Autodesk Fusion 360 part; units mm, degrees
(part 3 of 4)
  spline S28 degree 5 poles (-18.740221, -2.12836) (-18.744262, -2.124344) (-18.752452, -2.116435) (-18.765064, -2.104938) (-18.7825, -2.090307) (-18.805153, -2.072976) (-18.828436, -2.056341) (-18.852124, -2.040142) (-18.876048, -2.024187) (-18.90014, -2.008402) (-18.924398, -1.992794) (-18.948863, -1.977417) (-18.97359, -1.962339) (-18.998615, -1.947611) (-19.023939, -1.933234) (-19.049539, -1.919186) (-19.07538, -1.905425) (-19.101424, -1.891908) (-19.127643, -1.878606) (-19.154027, -1.865507) (-19.180576, -1.852613) (-19.207297, -1.839936) (-19.234197, -1.827485) (-19.261279, -1.815266) (-19.288542, -1.803279) (-19.315977, -1.791517) (-19.343576, -1.77997) (-19.37133, -1.768629) (-19.399233, -1.757488) (-19.427279, -1.746544) (-19.455469, -1.735796) (-19.4838, -1.725244) (-19.512273, -1.71489) (-19.540886, -1.704733) (-19.569636, -1.694772) (-19.598522, -1.685005) (-19.627539, -1.675429) (-19.656685, -1.666042) (-19.685956, -1.656842) (-19.71535, -1.647826) (-19.744866, -1.638995) (-19.774502, -1.630347) (-19.804256, -1.621883) (-19.834128, -1.613601) (-19.864114, -1.605501) (-19.894214, -1.597581) (-19.924425, -1.589841) (-19.954746, -1.582279) (-19.985174, -1.574894) (-20.015709, -1.567686) (-20.046348, -1.560654) (-20.077091, -1.553798) (-20.107936, -1.547117) (-20.138882, -1.540609) (-20.169926, -1.534276) (-20.201068, -1.528116) (-20.232307, -1.522128) (-20.26364, -1.516313) (-20.295067, -1.510669) (-20.326587, -1.505196) (-20.358197, -1.499894) (-20.389898, -1.494761) (-20.421688, -1.489799) (-20.453565, -1.485006) (-20.485528, -1.480381) (-20.517577, -1.475926) (-20.549708, -1.471638) (-20.581922, -1.467519) (-20.614218, -1.463567) (-20.646594, -1.459782) (-20.67905, -1.456164) (-20.705078, -1.453402) (-20.724635, -1.451406) (-20.737689, -1.450109) (-20.74422, -1.449468) knots 0 0 0 0 0 0 0.01428571 0.02857143 0.04285714 0.05714286 0.07142857 0.08571429 0.1 0.11428571 0.12857143 0.14285714 0.15714286 0.17142857 0.18571429 0.2 0.21428571 0.22857143 0.24285714 0.25714286 0.27142857 0.28571429 0.3 0.31428571 0.32857143 0.34285714 0.35714286 0.37142857 0.38571429 0.4 0.41428571 0.42857143 0.44285714 0.45714286 0.47142857 0.48571429 0.5 0.51428571 0.52857143 0.54285714 0.55714286 0.57142857 0.58571429 0.6 0.61428571 0.62857143 0.64285714 0.65714286 0.67142857 0.68571429 0.7 0.71428571 0.72857143 0.74285714 0.75714286 0.77142857 0.78571429 0.8 0.81428571 0.82857143 0.84285714 0.85714286 0.87142857 0.88571429 0.9 0.91428571 0.92857143 0.94285714 0.95714286 0.97142857 0.98571429 1 1 1 1 1 1
  arc A14 (-20.74422, -1.449468) -> (-21.063932, -1.847201) centre (-12.332883, -8.53815) ccw
  spline S29 degree 5 poles (-19.970136, -3.658422) (-19.974927, -3.655338) (-19.984412, -3.649039) (-19.998351, -3.639194) (-20.016388, -3.62531) (-20.038183, -3.606913) (-20.059434, -3.58775) (-20.080347, -3.568098) (-20.101071, -3.548162) (-20.121666, -3.528027) (-20.142123, -3.507691) (-20.1624, -3.487103) (-20.18244, -3.466195) (-20.202204, -3.444921) (-20.221688, -3.42328) (-20.240911, -3.401298) (-20.259905, -3.379019) (-20.278704, -3.35649) (-20.297331, -3.333743) (-20.315796, -3.310791) (-20.334094, -3.287634) (-20.352219, -3.264263) (-20.370162, -3.240669) (-20.387916, -3.216846) (-20.405483, -3.192797) (-20.422868, -3.168532) (-20.440078, -3.14406) (-20.457119, -3.119392) (-20.473997, -3.094537) (-20.490715, -3.069498) (-20.507271, -3.044278) (-20.523667, -3.018877) (-20.539899, -2.993296) (-20.555969, -2.967535) (-20.571877, -2.941598) (-20.587625, -2.915487) (-20.603214, -2.889206) (-20.618647, -2.86276) (-20.633925, -2.836151) (-20.649048, -2.809382) (-20.664017, -2.782454) (-20.678833, -2.75537) (-20.693495, -2.72813) (-20.708005, -2.700738) (-20.722361, -2.673193) (-20.736566, -2.6455) (-20.75062, -2.617659) (-20.764523, -2.589672) (-20.778276, -2.561543) (-20.791879, -2.533271) (-20.805332, -2.504859) (-20.818637, -2.476309) (-20.831792, -2.447621) (-20.844799, -2.418798) (-20.857658, -2.38984) (-20.870368, -2.36075) (-20.882931, -2.331529) (-20.895345, -2.302178) (-20.907613, -2.272699) (-20.919733, -2.243093) (-20.931707, -2.213361) (-20.943533, -2.183505) (-20.955213, -2.153525) (-20.966747, -2.123423) (-20.978134, -2.093201) (-20.989374, -2.06286) (-21.000468, -2.032401) (-21.011416, -2.001825) (-21.022218, -1.971134) (-21.032874, -1.940329) (-21.043384, -1.909409) (-21.051675, -1.884583) (-21.057829, -1.865912) (-21.061902, -1.853442) (-21.063932, -1.847201) knots 0 0 0 0 0 0 0.01428571 0.02857143 0.04285714 0.05714286 0.07142857 0.08571429 0.1 0.11428571 0.12857143 0.14285714 0.15714286 0.17142857 0.18571429 0.2 0.21428571 0.22857143 0.24285714 0.25714286 0.27142857 0.28571429 0.3 0.31428571 0.32857143 0.34285714 0.35714286 0.37142857 0.38571429 0.4 0.41428571 0.42857143 0.44285714 0.45714286 0.47142857 0.48571429 0.5 0.51428571 0.52857143 0.54285714 0.55714286 0.57142857 0.58571429 0.6 0.61428571 0.62857143 0.64285714 0.65714286 0.67142857 0.68571429 0.7 0.71428571 0.72857143 0.74285714 0.75714286 0.77142857 0.78571429 0.8 0.81428571 0.82857143 0.84285714 0.85714286 0.87142857 0.88571429 0.9 0.91428571 0.92857143 0.94285714 0.95714286 0.97142857 0.98571429 1 1 1 1 1 1
  line L29 (-19.970136, -3.658422) -> (-19.69789, -3.833648)
  line L30 (-20.118424, -4.568134) -> (-20.407357, -4.422054)
  spline S30 degree 5 poles (-20.407357, -4.422054) (-20.412442, -4.419483) (-20.422675, -4.414492) (-20.438222, -4.407455) (-20.459326, -4.398929) (-20.486226, -4.389446) (-20.51351, -4.380819) (-20.541045, -4.372733) (-20.568728, -4.364952) (-20.596518, -4.357385) (-20.624412, -4.350037) (-20.652432, -4.342972) (-20.680608, -4.336273) (-20.708959, -4.329999) (-20.737487, -4.324152) (-20.766175, -4.318702) (-20.795003, -4.313599) (-20.823949, -4.308793) (-20.852996, -4.304243) (-20.882136, -4.299938) (-20.91137, -4.29588) (-20.940701, -4.29208) (-20.970132, -4.288551) (-20.999665, -4.2853) (-21.029297, -4.282324) (-21.059024, -4.279615) (-21.088841, -4.277162) (-21.118741, -4.274953) (-21.14872, -4.27298) (-21.178777, -4.271238) (-21.208908, -4.269726) (-21.239113, -4.268446) (-21.269392, -4.267397) (-21.299743, -4.266579) (-21.330164, -4.265991) (-21.360655, -4.265628) (-21.391211, -4.265487) (-21.42183, -4.265566) (-21.452512, -4.265861) (-21.483254, -4.26637) (-21.514054, -4.267092) (-21.544911, -4.268026) (-21.575825, -4.269171) (-21.606794, -4.270525) (-21.637816, -4.272087) (-21.66889, -4.273856) (-21.700014, -4.27583) (-21.731187, -4.278008) (-21.762409, -4.280388) (-21.793676, -4.282969) (-21.824989, -4.285749) (-21.856346, -4.288728) (-21.887746, -4.291906) (-21.919188, -4.29528) (-21.95067, -4.29885) (-21.982192, -4.302614) (-22.013751, -4.306573) (-22.045348, -4.310725) (-22.076981, -4.315069) (-22.108649, -4.319604) (-22.140351, -4.324329) (-22.172086, -4.329244) (-22.203854, -4.334348) (-22.235652, -4.33964) (-22.26748, -4.345119) (-22.299336, -4.350785) (-22.33122, -4.356636) (-22.363131, -4.362673) (-22.395067, -4.368895) (-22.427028, -4.3753) (-22.459013, -4.381888) (-22.484621, -4.387305) (-22.503838, -4.39145) (-22.516654, -4.39425) (-22.523063, -4.395659) knots 0 0 0 0 0 0 0.01428571 0.02857143 0.04285714 0.05714286 0.07142857 0.08571429 0.1 0.11428571 0.12857143 0.14285714 0.15714286 0.17142857 0.18571429 0.2 0.21428571 0.22857143 0.24285714 0.25714286 0.27142857 0.28571429 0.3 0.31428571 0.32857143 0.34285714 0.35714286 0.37142857 0.38571429 0.4 0.41428571 0.42857143 0.44285714 0.45714286 0.47142857 0.48571429 0.5 0.51428571 0.52857143 0.54285714 0.55714286 0.57142857 0.58571429 0.6 0.61428571 0.62857143 0.64285714 0.65714286 0.67142857 0.68571429 0.7 0.71428571 0.72857143 0.74285714 0.75714286 0.77142857 0.78571429 0.8 0.81428571 0.82857143 0.84285714 0.85714286 0.87142857 0.88571429 0.9 0.91428571 0.92857143 0.94285714 0.95714286 0.97142857 0.98571429 1 1 1 1 1 1
  arc A15 (-22.523063, -4.395659) -> (-22.70422, -4.872722) centre (-12.332883, -8.53815) ccw
  spline S31 degree 5 poles (-21.104261, -6.257294) (-21.10977, -6.255842) (-21.120737, -6.252782) (-21.137036, -6.247726) (-21.158481, -6.240095) (-21.184895, -6.229333) (-21.211028, -6.217675) (-21.236989, -6.205447) (-21.26286, -6.192892) (-21.288668, -6.180106) (-21.314409, -6.167087) (-21.340056, -6.153773) (-21.365576, -6.140081) (-21.390946, -6.125956) (-21.416164, -6.111394) (-21.441239, -6.096428) (-21.466188, -6.081109) (-21.491029, -6.065492) (-21.515774, -6.049615) (-21.540427, -6.033492) (-21.564986, -6.017123) (-21.589446, -6.000497) (-21.613801, -5.983602) (-21.638048, -5.966431) (-21.662187, -5.948988) (-21.686219, -5.931282) (-21.710149, -5.913326) (-21.733979, -5.895132) (-21.757712, -5.876709) (-21.781348, -5.858062) (-21.804888, -5.839192) (-21.82833, -5.820101) (-21.851673, -5.800788) (-21.874917, -5.781254) (-21.898062, -5.761502) (-21.921108, -5.741535) (-21.944055, -5.721358) (-21.966905, -5.700975) (-21.989657, -5.68039) (-22.012312, -5.659604) (-22.03487, -5.63862) (-22.05733, -5.61744) (-22.079693, -5.596064) (-22.101957, -5.574496) (-22.124122, -5.552736) (-22.14619, -5.530788) (-22.168159, -5.508652) (-22.19003, -5.486332) (-22.211802, -5.463828) (-22.233475, -5.441144) (-22.25505, -5.41828) (-22.276526, -5.395238) (-22.297903, -5.37202) (-22.31918, -5.348627) (-22.340358, -5.32506) (-22.361435, -5.301322) (-22.382413, -5.277413) (-22.40329, -5.253335) (-22.424066, -5.229089) (-22.444742, -5.204678) (-22.465317, -5.180101) (-22.485791, -5.15536) (-22.506164, -5.130457) (-22.526435, -5.105393) (-22.546604, -5.080169) (-22.56667, -5.054786) (-22.586633, -5.029246) (-22.606494, -5.00355) (-22.626251, -4.977699) (-22.645905, -4.951694) (-22.665455, -4.925536) (-22.681013, -4.904486) (-22.692635, -4.888631) (-22.700362, -4.87803) (-22.70422, -4.872722) knots 0 0 0 0 0 0 0.01428571 0.02857143 0.04285714 0.05714286 0.07142857 0.08571429 0.1 0.11428571 0.12857143 0.14285714 0.15714286 0.17142857 0.18571429 0.2 0.21428571 0.22857143 0.24285714 0.25714286 0.27142857 0.28571429 0.3 0.31428571 0.32857143 0.34285714 0.35714286 0.37142857 0.38571429 0.4 0.41428571 0.42857143 0.44285714 0.45714286 0.47142857 0.48571429 0.5 0.51428571 0.52857143 0.54285714 0.55714286 0.57142857 0.58571429 0.6 0.61428571 0.62857143 0.64285714 0.65714286 0.67142857 0.68571429 0.7 0.71428571 0.72857143 0.74285714 0.75714286 0.77142857 0.78571429 0.8 0.81428571 0.82857143 0.84285714 0.85714286 0.87142857 0.88571429 0.9 0.91428571 0.92857143 0.94285714 0.95714286 0.97142857 0.98571429 1 1 1 1 1 1
  line L31 (-21.104261, -6.257294) -> (-20.791192, -6.339815)
  line L32 (-20.964175, -7.168305) -> (-21.284108, -7.11866)
  spline S32 degree 5 poles (-21.284108, -7.11866) (-21.289738, -7.117786) (-21.301013, -7.116202) (-21.317973, -7.114314) (-21.34068, -7.112726) (-21.369193, -7.112019) (-21.397807, -7.112246) (-21.426493, -7.113065) (-21.455226, -7.114219) (-21.483995, -7.11561) (-21.512794, -7.117241) (-21.541626, -7.119181) (-21.570492, -7.121517) (-21.599395, -7.12431) (-21.628333, -7.127565) (-21.657302, -7.131247) (-21.686296, -7.135303) (-21.71531, -7.139676) (-21.744341, -7.144325) (-21.773385, -7.149236) (-21.802443, -7.15441) (-21.831512, -7.15986) (-21.860593, -7.165598) (-21.889685, -7.171632) (-21.918786, -7.177959) (-21.947896, -7.184569) (-21.977011, -7.191449) (-22.006131, -7.198588) (-22.035253, -7.205975) (-22.064376, -7.213607) (-22.093499, -7.22148) (-22.122622, -7.229597) (-22.151743, -7.237956) (-22.180861, -7.246557) (-22.209976, -7.255398) (-22.239086, -7.264475) (-22.26819, -7.273784) (-22.297287, -7.283321) (-22.326375, -7.293082) (-22.355455, -7.303066) (-22.384525, -7.313271) (-22.413583, -7.323694) (-22.442631, -7.334335) (-22.471665, -7.345193) (-22.500686, -7.356265) (-22.529692, -7.36755) (-22.558683, -7.379046) (-22.587658, -7.39075) (-22.616616, -7.402661) (-22.645555, -7.414778) (-22.674477, -7.427099) (-22.703378, -7.439622) (-22.732259, -7.452347) (-22.76112, -7.465272) (-22.789958, -7.478395) (-22.818773, -7.491717) (-22.847565, -7.505234) (-22.876333, -7.518947) (-22.905075, -7.532853) (-22.933792, -7.546952) (-22.962482, -7.561242) (-22.991145, -7.575723) (-23.01978, -7.590394) (-23.048387, -7.605253) (-23.076964, -7.6203) (-23.10551, -7.635532) (-23.134026, -7.65095) (-23.162509, -7.666553) (-23.190959, -7.682338) (-23.219377, -7.698306) (-23.247761, -7.714456) (-23.270441, -7.727522) (-23.287437, -7.737402) (-23.29876, -7.744025) (-23.30442, -7.747346) knots 0 0 0 0 0 0 0.01428571 0.02857143 0.04285714 0.05714286 0.07142857 0.08571429 0.1 0.11428571 0.12857143 0.14285714 0.15714286 0.17142857 0.18571429 0.2 0.21428571 0.22857143 0.24285714 0.25714286 0.27142857 0.28571429 0.3 0.31428571 0.32857143 0.34285714 0.35714286 0.37142857 0.38571429 0.4 0.41428571 0.42857143 0.44285714 0.45714286 0.47142857 0.48571429 0.5 0.51428571 0.52857143 0.54285714 0.55714286 0.57142857 0.58571429 0.6 0.61428571 0.62857143 0.64285714 0.65714286 0.67142857 0.68571429 0.7 0.71428571 0.72857143 0.74285714 0.75714286 0.77142857 0.78571429 0.8 0.81428571 0.82857143 0.84285714 0.85714286 0.87142857 0.88571429 0.9 0.91428571 0.92857143 0.94285714 0.95714286 0.97142857 0.98571429 1 1 1 1 1 1
  arc A16 (-23.30442, -7.747346) -> (-23.329291, -8.25704) centre (-12.332883, -8.53815) ccw
  spline S33 degree 5 poles (-21.379783, -9.079432) (-21.385471, -9.079753) (-21.396847, -9.080232) (-21.41391, -9.08046) (-21.436663, -9.07983) (-21.46511, -9.077757) (-21.493566, -9.074745) (-21.522036, -9.071138) (-21.55052, -9.067192) (-21.579017, -9.063007) (-21.607521, -9.058579) (-21.636026, -9.053842) (-21.664528, -9.048707) (-21.693022, -9.043112) (-21.721506, -9.037056) (-21.749978, -9.030571) (-21.778439, -9.023712) (-21.80689, -9.016535) (-21.835331, -9.009081) (-21.863759, -9.001366) (-21.892175, -8.993387) (-21.920575, -8.985134) (-21.948959, -8.976591) (-21.977326, -8.967754) (-22.005673, -8.958624) (-22.034001, -8.949211) (-22.062308, -8.939529) (-22.090594, -8.929589) (-22.118858, -8.919401) (-22.1471, -8.908971) (-22.175319, -8.898299) (-22.203513, -8.887386) (-22.231682, -8.876232) (-22.259824, -8.864837) (-22.28794, -8.853203) (-22.316028, -8.841335) (-22.344087, -8.829237) (-22.372117, -8.816913) (-22.400118, -8.804366) (-22.428087, -8.791598) (-22.456025, -8.778612) (-22.483931, -8.765409) (-22.511804, -8.75199) (-22.539644, -8.738357) (-22.567449, -8.724512) (-22.595218, -8.710457) (-22.622953, -8.696193) (-22.65065, -8.681724) (-22.678311, -8.66705) (-22.705933, -8.652173) (-22.733518, -8.637096) (-22.761063, -8.621818) (-22.788568, -8.606342) (-22.816033, -8.590669) (-22.843456, -8.5748) (-22.870838, -8.558736) (-22.898177, -8.54248) (-22.925473, -8.526032) (-22.952725, -8.509393) (-22.979932, -8.492566) (-23.007095, -8.47555) (-23.034212, -8.458347) (-23.061283, -8.440958) (-23.088307, -8.423385) (-23.115283, -8.405627) (-23.142211, -8.387688) (-23.16909, -8.369567) (-23.195919, -8.351266) (-23.222697, -8.332785) (-23.249425, -8.314127) (-23.276102, -8.29529) (-23.297403, -8.280078) (-23.313356, -8.26859) (-23.323981, -8.260896) (-23.329291, -8.25704) knots 0 0 0 0 0 0 0.01428571 0.02857143 0.04285714 0.05714286 0.07142857 0.08571429 0.1 0.11428571 0.12857143 0.14285714 0.15714286 0.17142857 0.18571429 0.2 0.21428571 0.22857143 0.24285714 0.25714286 0.27142857 0.28571429 0.3 0.31428571 0.32857143 0.34285714 0.35714286 0.37142857 0.38571429 0.4 0.41428571 0.42857143 0.44285714 0.45714286 0.47142857 0.48571429 0.5 0.51428571 0.52857143 0.54285714 0.55714286 0.57142857 0.58571429 0.6 0.61428571 0.62857143 0.64285714 0.65714286 0.67142857 0.68571429 0.7 0.71428571 0.72857143 0.74285714 0.75714286 0.77142857 0.78571429 0.8 0.81428571 0.82857143 0.84285714 0.85714286 0.87142857 0.88571429 0.9 0.91428571 0.92857143 0.94285714 0.95714286 0.97142857 0.98571429 1 1 1 1 1 1
  line L33 (-21.379783, -9.079432) -> (-21.056536, -9.06117)
  line L34 (-20.965034, -9.902566) -> (-21.284651, -9.954215)
  spline S34 degree 5 poles (-21.284651, -9.954215) (-21.290275, -9.955124) (-21.301487, -9.957101) (-21.318201, -9.960547) (-21.340287, -9.966053) (-21.367623, -9.974192) (-21.394767, -9.983251) (-21.421796, -9.992893) (-21.448766, -10.00287) (-21.475696, -10.013083) (-21.502582, -10.023534) (-21.529403, -10.034288) (-21.556135, -10.04543) (-21.58276, -10.057018) (-21.609276, -10.069056) (-21.635689, -10.081509) (-21.662011, -10.094326) (-21.688254, -10.107451) (-21.714427, -10.120844) (-21.740532, -10.13449) (-21.766569, -10.14839) (-21.792531, -10.162556) (-21.818416, -10.177) (-21.844219, -10.191728) (-21.869941, -10.206738) (-21.895583, -10.22202) (-21.921147, -10.237561) (-21.946636, -10.253349) (-21.972049, -10.269374) (-21.997389, -10.285631) (-22.022654, -10.302119) (-22.047843, -10.318837) (-22.072956, -10.335786) (-22.097991, -10.352965) (-22.122949, -10.37037) (-22.147829, -10.387998) (-22.172632, -10.405845) (-22.197357, -10.423906) (-22.222006, -10.442179) (-22.246577, -10.46066) (-22.271071, -10.479348) (-22.295486, -10.498242) (-22.319823, -10.517338) (-22.344081, -10.536637) (-22.36826, -10.556135) (-22.39236, -10.575831) (-22.41638, -10.595722) (-22.440319, -10.615807) (-22.464179, -10.636084) (-22.487958, -10.656551) (-22.511657, -10.677205) (-22.535274, -10.698047) (-22.558809, -10.719074) (-22.582263, -10.740284) (-22.605634, -10.761677) (-22.628923, -10.783251) (-22.652128, -10.805004) (-22.67525, -10.826935) (-22.698289, -10.849042) (-22.721243, -10.871325) (-22.744113, -10.893782) (-22.766899, -10.916412) (-22.789599, -10.939213) (-22.812214, -10.962185) (-22.834742, -10.985326) (-22.857185, -11.008635) (-22.87954, -11.03211) (-22.901808, -11.05575) (-22.923987, -11.079555) (-22.94608, -11.103523) (-22.968084, -11.127653) (-22.985617, -11.147088) (-22.998727, -11.161737) (-23.00745, -11.171535) (-23.011807, -11.176442) knots 0 0 0 0 0 0 0.01428571 0.02857143 0.04285714 0.05714286 0.07142857 0.08571429 0.1 0.11428571 0.12857143 0.14285714 0.15714286 0.17142857 0.18571429 0.2 0.21428571 0.22857143 0.24285714 0.25714286 0.27142857 0.28571429 0.3 0.31428571 0.32857143 0.34285714 0.35714286 0.37142857 0.38571429 0.4 0.41428571 0.42857143 0.44285714 0.45714286 0.47142857 0.48571429 0.5 0.51428571 0.52857143 0.54285714 0.55714286 0.57142857 0.58571429 0.6 0.61428571 0.62857143 0.64285714 0.65714286 0.67142857 0.68571429 0.7 0.71428571 0.72857143 0.74285714 0.75714286 0.77142857 0.78571429 0.8 0.81428571 0.82857143 0.84285714 0.85714286 0.87142857 0.88571429 0.9 0.91428571 0.92857143 0.94285714 0.95714286 0.97142857 0.98571429 1 1 1 1 1 1
  arc A17 (-23.011807, -11.176442) -> (-22.877956, -11.668875) centre (-12.332883, -8.53815) ccw
  spline S35 degree 5 poles (-20.769731, -11.848585) (-20.775041, -11.850648) (-20.785712, -11.854619) (-20.80187, -11.860109) (-20.823704, -11.866541) (-20.851399, -11.87336) (-20.879394, -11.879289) (-20.907585, -11.884656) (-20.935894, -11.889705) (-20.964289, -11.894531) (-20.992766, -11.899128) (-21.021341, -11.903431) (-21.050034, -11.907355) (-21.078862, -11.91084) (-21.107823, -11.913882) (-21.136906, -11.916513) (-21.166094, -11.918784) (-21.19537, -11.92075) (-21.224722, -11.92245) (-21.254143, -11.923897) (-21.283633, -11.92509) (-21.313195, -11.926016) (-21.342829, -11.926664) (-21.372538, -11.927024) (-21.402319, -11.927101) (-21.432169, -11.926903) (-21.462083, -11.926441) (-21.492056, -11.925729) (-21.522085, -11.924774) (-21.552168, -11.923582) (-21.582303, -11.922152) (-21.61249, -11.920486) (-21.642727, -11.918582) (-21.673014, -11.916441) (-21.703348, -11.914065) (-21.733728, -11.911458) (-21.764153, -11.908623) (-21.79462, -11.905563) (-21.825127, -11.902283) (-21.855673, -11.898783) (-21.886256, -11.895066) (-21.916877, -11.891132) (-21.947532, -11.886983) (-21.978222, -11.882621) (-22.008944, -11.878046) (-22.039698, -11.87326) (-22.070483, -11.868265) (-22.101296, -11.863062) (-22.132137, -11.857654) (-22.163005, -11.852042) (-22.193898, -11.846226) (-22.224816, -11.840208) (-22.255758, -11.833989) (-22.286722, -11.82757) (-22.317707, -11.820952) (-22.348712, -11.814136) (-22.379736, -11.807123) (-22.410779, -11.799915) (-22.441839, -11.792512) (-22.472915, -11.784916) (-22.504006, -11.777127) (-22.535112, -11.769145) (-22.566231, -11.760973) (-22.597363, -11.75261) (-22.628507, -11.744058) (-22.659661, -11.735318) (-22.690823, -11.72639) (-22.721995, -11.717275) (-22.753173, -11.707974) (-22.784359, -11.698488) (-22.815551, -11.688817) (-22.84051, -11.680932) (-22.859232, -11.674936) (-22.871714, -11.670902) (-22.877956, -11.668875) knots 0 0 0 0 0 0 0.01428571 0.02857143 0.04285714 0.05714286 0.07142857 0.08571429 0.1 0.11428571 0.12857143 0.14285714 0.15714286 0.17142857 0.18571429 0.2 0.21428571 0.22857143 0.24285714 0.25714286 0.27142857 0.28571429 0.3 0.31428571 0.32857143 0.34285714 0.35714286 0.37142857 0.38571429 0.4 0.41428571 0.42857143 0.44285714 0.45714286 0.47142857 0.48571429 0.5 0.51428571 0.52857143 0.54285714 0.55714286 0.57142857 0.58571429 0.6 0.61428571 0.62857143 0.64285714 0.65714286 0.67142857 0.68571429 0.7 0.71428571 0.72857143 0.74285714 0.75714286 0.77142857 0.78571429 0.8 0.81428571 0.82857143 0.84285714 0.85714286 0.87142857 0.88571429 0.9 0.91428571 0.92857143 0.94285714 0.95714286 0.97142857 0.98571429 1 1 1 1 1 1
  line L35 (-20.769731, -11.848585) -> (-20.467948, -11.731329)
  line L36 (-20.120919, -12.503268) -> (-20.408932, -12.651156)
  spline S36 degree 5 poles (-20.408932, -12.651156) (-20.413999, -12.653758) (-20.424053, -12.659104) (-20.438884, -12.667546) (-20.458187, -12.679607) (-20.48167, -12.695796) (-20.504686, -12.712798) (-20.527412, -12.730321) (-20.549979, -12.748144) (-20.572436, -12.766179) (-20.594776, -12.784427) (-20.616961, -12.802943) (-20.638942, -12.8218) (-20.660683, -12.841049) (-20.682181, -12.860691) (-20.703453, -12.880697) (-20.724526, -12.901021) (-20.745428, -12.921613) (-20.766182, -12.942438) (-20.786793, -12.963483) (-20.807259, -12.984748) (-20.827574, -13.006244) (-20.847728, -13.027979) (-20.867717, -13.049961) (-20.887542, -13.072185) (-20.907207, -13.094642) (-20.926717, -13.117323) (-20.946079, -13.140214) (-20.965297, -13.163308) (-20.984373, -13.1866) (-21.003306, -13.210088) (-21.022097, -13.233772) (-21.040743, -13.257652) (-21.059244, -13.281726) (-21.077602, -13.305991) (-21.095817, -13.330445) (-21.113891, -13.355083) (-21.131825, -13.379901) (-21.149621, -13.404896) (-21.167278, -13.430066) (-21.184798, -13.455408) (-21.20218, -13.480922) (-21.219425, -13.506604) (-21.236532, -13.532454) (-21.253502, -13.55847) (-21.270336, -13.584649) (-21.287033, -13.610989) (-21.303595, -13.637489) (-21.320021, -13.664147) (-21.336312, -13.69096) (-21.352467, -13.717927) (-21.368488, -13.745046) (-21.384374, -13.772317) (-21.400126, -13.799737) (-21.415742, -13.827305) (-21.431224, -13.855019) (-21.446572, -13.882878) (-21.461785, -13.910881) (-21.476865, -13.939026) (-21.49181, -13.967311) (-21.506621, -13.995736) (-21.521298, -14.024299) (-21.535841, -14.053) (-21.550251, -14.081836) (-21.564526, -14.110806) (-21.578667, -14.139908) (-21.592674, -14.169143) (-21.606546, -14.198507) (-21.620285, -14.228001) (-21.633889, -14.257622) (-21.647359, -14.287372) (-21.658029, -14.311273) (-21.665971, -14.329256) (-21.671239, -14.34127) (-21.673866, -14.347284) knots 0 0 0 0 0 0 0.01428571 0.02857143 0.04285714 0.05714286 0.07142857 0.08571429 0.1 0.11428571 0.12857143 0.14285714 0.15714286 0.17142857 0.18571429 0.2 0.21428571 0.22857143 0.24285714 0.25714286 0.27142857 0.28571429 0.3 0.31428571 0.32857143 0.34285714 0.35714286 0.37142857 0.38571429 0.4 0.41428571 0.42857143 0.44285714 0.45714286 0.47142857 0.48571429 0.5 0.51428571 0.52857143 0.54285714 0.55714286 0.57142857 0.58571429 0.6 0.61428571 0.62857143 0.64285714 0.65714286 0.67142857 0.68571429 0.7 0.71428571 0.72857143 0.74285714 0.75714286 0.77142857 0.78571429 0.8 0.81428571 0.82857143 0.84285714 0.85714286 0.87142857 0.88571429 0.9 0.91428571 0.92857143 0.94285714 0.95714286 0.97142857 0.98571429 1 1 1 1 1 1
  arc A18 (-21.673866, -14.347284) -> (-21.394396, -14.774253) centre (-12.332883, -8.53815) ccw
  spline S37 degree 5 poles (-19.333821, -14.29369) (-19.338234, -14.297293) (-19.347156, -14.304368) (-19.360827, -14.314582) (-19.379605, -14.327446) (-19.403837, -14.342489) (-19.428629, -14.356779) (-19.453782, -14.370595) (-19.479145, -14.384145) (-19.504659, -14.397509) (-19.530322, -14.410681) (-19.556168, -14.423604) (-19.582245, -14.436202) (-19.608585, -14.448425) (-19.635189, -14.460267) (-19.662035, -14.471757) (-19.689093, -14.482936) (-19.716328, -14.493853) (-19.743718, -14.50454) (-19.771252, -14.515008) (-19.79893, -14.525255) (-19.826759, -14.535271) (-19.854743, -14.545044) (-19.882886, -14.554568) (-19.911186, -14.563844) (-19.939636, -14.572879) (-19.968228, -14.581684) (-19.996955, -14.590269) (-20.025809, -14.598641) (-20.054788, -14.606803) (-20.08389, -14.614755) (-20.113114, -14.622499) (-20.14246, -14.630032) (-20.171926, -14.637355) (-20.20151, -14.644469) (-20.231209, -14.651377) (-20.26102, -14.658083) (-20.290941, -14.664588) (-20.320969, -14.670895) (-20.351102, -14.677006) (-20.381337, -14.682921) (-20.411674, -14.688642) (-20.442111, -14.69417) (-20.472647, -14.699504) (-20.503279, -14.704647) (-20.534007, -14.709598) (-20.564828, -14.714361) (-20.595741, -14.718935) (-20.626744, -14.723322) (-20.657836, -14.727523) (-20.689014, -14.731538) (-20.720279, -14.735369) (-20.751627, -14.739016) (-20.783059, -14.742479) (-20.814573, -14.74576) (-20.846167, -14.748859) (-20.87784, -14.751777) (-20.909591, -14.754514) (-20.941418, -14.757072) (-20.97332, -14.75945) (-21.005297, -14.76165) (-21.037347, -14.763671) (-21.069469, -14.765515) (-21.101661, -14.767182) (-21.133923, -14.768673) (-21.166253, -14.769987) (-21.198649, -14.771126) (-21.231111, -14.77209) (-21.263638, -14.772879) (-21.296229, -14.773494) (-21.328883, -14.773935) (-21.355056, -14.774149) (-21.374715, -14.774231) (-21.387833, -14.774252) (-21.394396, -14.774253) knots 0 0 0 0 0 0 0.01428571 0.02857143 0.04285714 0.05714286 0.07142857 0.08571429 0.1 0.11428571 0.12857143 0.14285714 0.15714286 0.17142857 0.18571429 0.2 0.21428571 0.22857143 0.24285714 0.25714286 0.27142857 0.28571429 0.3 0.31428571 0.32857143 0.34285714 0.35714286 0.37142857 0.38571429 0.4 0.41428571 0.42857143 0.44285714 0.45714286 0.47142857 0.48571429 0.5 0.51428571 0.52857143 0.54285714 0.55714286 0.57142857 0.58571429 0.6 0.61428571 0.62857143 0.64285714 0.65714286 0.67142857 0.68571429 0.7 0.71428571 0.72857143 0.74285714 0.75714286 0.77142857 0.78571429 0.8 0.81428571 0.82857143 0.84285714 0.85714286 0.87142857 0.88571429 0.9 0.91428571 0.92857143 0.94285714 0.95714286 0.97142857 0.98571429 1 1 1 1 1 1
  line L37 (-19.333821, -14.29369) -> (-19.083043, -14.088917)
  line L38 (-18.514457, -14.715837) -> (-18.742673, -14.945488)
  spline S38 degree 5 poles (-18.742673, -14.945488) (-18.746688, -14.949529) (-18.754598, -14.957719) (-18.766094, -14.970331) (-18.780725, -14.987767) (-18.798056, -15.01042) (-18.814692, -15.033703) (-18.830891, -15.057391) (-18.846846, -15.081315) (-18.862631, -15.105406) (-18.878239, -15.129665) (-18.893616, -15.15413) (-18.908694, -15.178856) (-18.923422, -15.203882) (-18.937799, -15.229206) (-18.951847, -15.254806) (-18.965608, -15.280647) (-18.979125, -15.30669) (-18.992427, -15.332909) (-19.005526, -15.359293) (-19.018419, -15.385843) (-19.031097, -15.412563) (-19.043548, -15.439463) (-19.055766, -15.466546) (-19.067753, -15.493808) (-19.079516, -15.521243) (-19.091063, -15.548843) (-19.102403, -15.576597) (-19.113545, -15.604499) (-19.124489, -15.632546) (-19.135237, -15.660735) (-19.145789, -15.689067) (-19.156143, -15.717539) (-19.1663, -15.746152) (-19.176261, -15.774903) (-19.186028, -15.803789) (-19.195604, -15.832806) (-19.204991, -15.861951) (-19.214191, -15.891222) (-19.223207, -15.920617) (-19.232038, -15.950133) (-19.240685, -15.979769) (-19.24915, -16.009523) (-19.257432, -16.039394) (-19.265532, -16.069381) (-19.273452, -16.09948) (-19.281192, -16.129692) (-19.288754, -16.160012) (-19.296139, -16.190441) (-19.303347, -16.220975) (-19.310379, -16.251615) (-19.317235, -16.282358) (-19.323916, -16.313203) (-19.330423, -16.344148) (-19.336757, -16.375193) (-19.342917, -16.406335) (-19.348904, -16.437574) (-19.35472, -16.468907) (-19.360364, -16.500334) (-19.365837, -16.531853) (-19.371139, -16.563464) (-19.376272, -16.595165) (-19.381234, -16.626954) (-19.386027, -16.658831) (-19.390652, -16.690795) (-19.395107, -16.722843) (-19.399395, -16.754975) (-19.403514, -16.787189) (-19.407466, -16.819484) (-19.411251, -16.85186) (-19.414869, -16.884316) (-19.41763, -16.910345) (-19.419627, -16.929902) (-19.420924, -16.942956) (-19.421565, -16.949487) knots 0 0 0 0 0 0 0.01428571 0.02857143 0.04285714 0.05714286 0.07142857 0.08571429 0.1 0.11428571 0.12857143 0.14285714 0.15714286 0.17142857 0.18571429 0.2 0.21428571 0.22857143 0.24285714 0.25714286 0.27142857 0.28571429 0.3 0.31428571 0.32857143 0.34285714 0.35714286 0.37142857 0.38571429 0.4 0.41428571 0.42857143 0.44285714 0.45714286 0.47142857 0.48571429 0.5 0.51428571 0.52857143 0.54285714 0.55714286 0.57142857 0.58571429 0.6 0.61428571 0.62857143 0.64285714 0.65714286 0.67142857 0.68571429 0.7 0.71428571 0.72857143 0.74285714 0.75714286 0.77142857 0.78571429 0.8 0.81428571 0.82857143 0.84285714 0.85714286 0.87142857 0.88571429 0.9 0.91428571 0.92857143 0.94285714 0.95714286 0.97142857 0.98571429 1 1 1 1 1 1
  arc A19 (-19.421565, -16.949487) -> (-19.023832, -17.269198) centre (-12.332883, -8.53815) ccw
  spline S39 degree 5 poles (-17.212611, -16.175403) (-17.215694, -16.180193) (-17.221993, -16.189678) (-17.231839, -16.203617) (-17.245723, -16.221654) (-17.26412, -16.243449) (-17.283283, -16.264701) (-17.302935, -16.285613) (-17.322871, -16.306338) (-17.343006, -16.326932) (-17.363342, -16.34739) (-17.38393, -16.367667) (-17.404837, -16.387707) (-17.426112, -16.407471) (-17.447753, -16.426955) (-17.469735, -16.446178) (-17.492014, -16.465172) (-17.514543, -16.48397) (-17.53729, -16.502598) (-17.560242, -16.521062) (-17.583399, -16.539361) (-17.60677, -16.557486) (-17.630364, -16.575428) (-17.654187, -16.593183) (-17.678236, -16.61075) (-17.702501, -16.628135) (-17.726973, -16.645344) (-17.751641, -16.662386) (-17.776496, -16.679264) (-17.801535, -16.695981) (-17.826755, -16.712538) (-17.852155, -16.728933) (-17.877737, -16.745166) (-17.903498, -16.761236) (-17.929435, -16.777144) (-17.955546, -16.792892) (-17.981827, -16.808481) (-18.008273, -16.823914) (-18.034882, -16.839191) (-18.061651, -16.854314) (-18.088579, -16.869284) (-18.115663, -16.8841) (-18.142902, -16.898762) (-18.170295, -16.913271) (-18.197839, -16.927628) (-18.225533, -16.941833) (-18.253374, -16.955887) (-18.281361, -16.969789) (-18.30949, -16.983542) (-18.337762, -16.997145) (-18.366174, -17.010599) (-18.394724, -17.023903) (-18.423412, -17.037059) (-18.452235, -17.050066) (-18.481193, -17.062924) (-18.510283, -17.075635) (-18.539504, -17.088197) (-18.568855, -17.100612) (-18.598334, -17.11288) (-18.62794, -17.125) (-18.657672, -17.136973) (-18.687528, -17.1488) (-18.717508, -17.16048) (-18.74761, -17.172013) (-18.777832, -17.1834) (-18.808173, -17.194641) (-18.838632, -17.205735) (-18.869208, -17.216683) (-18.899899, -17.227484) (-18.930704, -17.23814) (-18.961624, -17.24865) (-18.98645, -17.256942) (-19.005121, -17.263096) (-19.017591, -17.267169) (-19.023832, -17.269198) knots 0 0 0 0 0 0 0.01428571 0.02857143 0.04285714 0.05714286 0.07142857 0.08571429 0.1 0.11428571 0.12857143 0.14285714 0.15714286 0.17142857 0.18571429 0.2 0.21428571 0.22857143 0.24285714 0.25714286 0.27142857 0.28571429 0.3 0.31428571 0.32857143 0.34285714 0.35714286 0.37142857 0.38571429 0.4 0.41428571 0.42857143 0.44285714 0.45714286 0.47142857 0.48571429 0.5 0.51428571 0.52857143 0.54285714 0.55714286 0.57142857 0.58571429 0.6 0.61428571 0.62857143 0.64285714 0.65714286 0.67142857 0.68571429 0.7 0.71428571 0.72857143 0.74285714 0.75714286 0.77142857 0.78571429 0.8 0.81428571 0.82857143 0.84285714 0.85714286 0.87142857 0.88571429 0.9 0.91428571 0.92857143 0.94285714 0.95714286 0.97142857 0.98571429 1 1 1 1 1 1
  line L39 (-17.212611, -16.175403) -> (-17.037385, -15.903157)
  circle A20 centre (-12.332883, -8.53815) radius 7.288702
  circle A21 centre (-12.332883, -8.53815) radius 2.585976
  line L40 (-19.69789, -3.833648) -> (-18.51057, -2.356576)
  line L41 (-20.467948, -11.731329) -> (-20.965034, -9.902566)
  line L42 (-20.791192, -6.339815) -> (-20.118424, -4.568134)
  line L43 (-19.083043, -14.088917) -> (-20.120919, -12.503268)
  line L44 (-21.056536, -9.06117) -> (-20.964175, -7.168305)
  line L45 (-4.197818, -5.344971) -> (-3.700732, -7.173734)
  line L46 (-3.874574, -10.736485) -> (-4.547342, -12.508165)
  line L47 (-17.88365, -1.78799) -> (-16.298001, -0.750114)
  line L48 (-5.582723, -2.987383) -> (-4.544847, -4.573032)
  line L49 (-15.526062, -0.403085) -> (-13.697299, 0.094002)
  line L50 (-12.855903, 0.185503) -> (-10.963038, 0.093142)
  line L51 (-10.134548, -0.079841) -> (-8.362867, -0.752609)
  line L52 (-7.628381, -1.173143) -> (-6.151309, -2.360463)
  line L53 (-11.809863, -17.261803) -> (-13.702728, -17.169441)
  line L54 (-3.60923, -8.015129) -> (-3.701592, -9.907995)
  line L55 (-4.967876, -13.242652) -> (-6.155196, -14.719723)
  line L56 (-6.782116, -15.288309) -> (-8.367765, -16.326186)
  line L57 (-9.139704, -16.673214) -> (-10.968467, -17.170301)
  line L58 (-14.531218, -16.996459) -> (-16.302899, -16.32369)
  line L59 (-17.037385, -15.903157) -> (-18.514457, -14.715837)
  constraint concentric A20 A21
extrude "Extruir3" add sketch "Boceto5" along normal blind 15 contours A20 picked at (-6.64852, -9.028731) sketch seen with x (0.8367022, 0.54765814, 0) y (0.54765814, -0.8367022, 0) z (0, 0, -1) at (-14.994937, 0.389685, 4) bodies 3 2 in component "Spur Gear (20 teeth) (1)"
sketch "Boceto6" plane through (0, 0, 19) normal (0, 0, 1) x (-1, 0, 0)
  circle A0 centre (-12.332883, -8.538149) radius 2.585976
  circle A1 centre (-12.332883, -8.538149) radius 7.288702
  circle A2 centre (-17.329868, -11.762187) radius 1.846918
extrude "Extruir4" cut sketch "Boceto6" against normal up to surface (15 mm away) contours A1 A2 picked at (-17.555212, -11.908939) sketch seen with x (0.99865804, -0.05178923, 0) y (-0.05178923, -0.99865804, 0) z (0, 0, -1) at (-11.874148, 9.165402, 4) bodies 2 3 in component "Spur Gear (20 teeth) (1)"
sketch "Boceto7" plane through (0, 0, 0) normal (0, 1, 0) x (1, 0, 0)
sketch "Boceto8" plane through (0, 0, 12) normal (0, 0, 1) x (-1, 0, 0)
  circle A0 centre (-12.332883, -8.53815) radius 2
  circle A1 centre (-12.332883, -8.53815) radius 0.772296
  constraint concentric A0 A1
extrude "Extruir3'" cut sketch "Boceto8" against normal blind 14 contours A1 picked at (-12.144172, -8.211292) bodies 24
ref_plane "PlanoDeObra2" through (14.525165, 9.909709, 11.280091) normal (-0.84775786, -0.53038346, 0) x (-0.53038346, 0.84775786, 0)
sketch "Boceto9" plane through (14.894909, 9.318714, 0) normal (-0.84775786, -0.53038346, 0) x (-0.53038346, 0.84775786, 0)
  circle A0 centre (0.54438, -11.557601) radius 1.123634
extrude "Extruir5" cut sketch "Boceto9" along normal mid plane 6 contours A0 picked at (0.186475, -10.937691) sketch seen with x (0.99865804, -0.05178923, 0) y (-0.05178923, -0.99865804, 0) z (0, 0, -1) at (-11.874148, 9.165402, 4) bodies 2 3 in component "Spur Gear (20 teeth) (1)"
sketch "Boceto10" plane through (0, 0, 19) normal (0, 0, 1) x (-1, -0.00000001, 0)
  arc A0 (-14.531455, -15.487355) -> (-16.986536, -14.147845) centre (-15.181128, -13.758473) ccw
  arc A1 (-14.531455, -15.487355) -> (-16.986536, -14.147845) centre (-12.332883, -8.538149) ccw
  circle A2 centre (-12.332883, -8.538149) radius 2.585976
  line L0 (-7.774405, -12.329513) -> (-6.725658, -12.329513)
  line L1 (-6.725658, -12.329513) -> (-6.725658, -13.19478)
  line L2 (-6.725658, -13.19478) -> (-7.774405, -13.19478)
  line L3 (-7.774405, -13.19478) -> (-7.774405, -12.329513)
  line L4 (-12.332883, -3.518559) -> (-12.332883, -13)
  line L5 (-19.178964, -8.538149) -> (-6, -8.538149)
  line L6 (-16.905658, -13.19478) -> (-17.954405, -13.19478)
  line L7 (-17.954405, -13.19478) -> (-17.954405, -12.329513)
  line L8 (-17.954405, -12.329513) -> (-16.905658, -12.329513)
  line L9 (-16.905658, -12.329513) -> (-16.905658, -13.19478)
  line L10 (-6.725658, -4.69478) -> (-7.774405, -4.69478)
  line L11 (-7.774405, -4.69478) -> (-7.774405, -3.829513)
  line L12 (-7.774405, -3.829513) -> (-6.725658, -3.829513)
  line L13 (-6.725658, -3.829513) -> (-6.725658, -4.69478)
  line L14 (-16.905658, -4.69478) -> (-17.954405, -4.69478)
  line L15 (-17.954405, -4.69478) -> (-17.954405, -3.829513)
  line L16 (-17.954405, -3.829513) -> (-16.905658, -3.829513)
  line L17 (-16.905658, -3.829513) -> (-16.905658, -4.69478)
  line L18 (-17.954405, -8.829513) -> (-16.905658, -8.829513)
  line L19 (-17.954405, -9.69478) -> (-17.954405, -8.829513)
  line L20 (-16.905658, -8.829513) -> (-16.905658, -9.69478)
  line L21 (-16.905658, -9.69478) -> (-17.954405, -9.69478)
  line L22 (-7.774405, -9.69478) -> (-7.774405, -8.829513)
  line L23 (-6.725658, -9.69478) -> (-7.774405, -9.69478)
  line L24 (-6.725658, -8.829513) -> (-6.725658, -9.69478)
  line L25 (-7.774405, -8.829513) -> (-6.725658, -8.829513)
  line L26 (-17.954405, -4.746785) -> (-16.905658, -4.746785)
  line L27 (-17.954405, -8.246785) -> (-16.905658, -8.246785)
  line L28 (-16.905658, -7.381519) -> (-17.954405, -7.381519)
  line L29 (-16.905658, -3.881519) -> (-17.954405, -3.881519)
  line L30 (-17.954405, -7.381519) -> (-17.954405, -8.246785)
  line L31 (-16.905658, -8.246785) -> (-16.905658, -7.381519)
  line L32 (-6.725658, -7.381519) -> (-7.774405, -7.381519)
  line L33 (-7.774405, -7.381519) -> (-7.774405, -8.246785)
  line L34 (-7.774405, -8.246785) -> (-6.725658, -8.246785)
  line L35 (-6.725658, -8.246785) -> (-6.725658, -7.381519)
  line L36 (-7.774405, -4.746785) -> (-6.725658, -4.746785)
  line L37 (-7.774405, -3.881519) -> (-7.774405, -4.746785)
  line L38 (-6.725658, -4.746785) -> (-6.725658, -3.881519)
  line L39 (-6.725658, -3.881519) -> (-7.774405, -3.881519)
  dimension "d170" = -10.18
  dimension "d171" = 8.5
  dimension "d174" = 0
  dimension "d175" = 3.5
  constraint horizontal L0
  constraint vertical L1
  constraint horizontal L2
  constraint vertical L3
  constraint vertical L4
  constraint horizontal L5
extrude "Extruir6" add sketch "Boceto10" along normal blind 1.5 contours L0 L1 L2 L3 | A0 A1 L6 L7 L8 L9 | L10 L11 L13 L37 L38 L39 | A1 L14 L15 L17 L29 | L18 L19 L20 L21 | L22 L23 L24 L25 | L27 L28 L30 L31 | L32 L33 L34 L35 picked at (-7.07524, -12.906357) picked at (-17.604823, -12.868119) picked at (-7.424823, -4.152606) picked at (-17.600057, -4.423693) picked at (-17.604823, -9.406357) picked at (-7.07524, -9.117935) picked at (-17.604823, -7.669941) picked at (-7.424823, -7.669941) sketch seen with x (0.90195158, 0.43183717, 0) y (0.43183717, -0.90195158, 0) z (0, 0, -1) at (-14.810754, 2.3752, 4) bodies 2 in component "Spur Gear (20 teeth) (1)"
sketch "Boceto11" plane through (0, 13.19478, 0) normal (-0.00000002, 1, 0) x (-1, -0.00000002, 0)
  line L0 (-17.940108, 19) -> (-16.939922, 19)
  line L1 (-16.939922, 19) -> (-16.939922, 20.5)
  line L2 (-16.939922, 20.5) -> (-17.940108, 20.5)
  line L3 (-17.940108, 20.5) -> (-17.940108, 19)
  circle A0 centre (-17.4, 20) radius 0.360555
sketch "Boceto1 (4)" plane through (0, 0, 0) normal (0, 0, 1) x (1, 0, 0) in component "Component"
  line L0 (1.875, 3.247595) -> (3.75, 0)
  line L1 (-1.875, 3.247595) -> (1.875, 3.247595)
  line L2 (-3.75, 0) -> (-1.875, 3.247595)
  line L3 (-1.875, -3.247595) -> (-3.75, 0)
  line L4 (1.875, -3.247595) -> (-1.875, -3.247595)
  line L5 (3.75, 0) -> (1.875, -3.247595)
extrude "Extruir1''''" add sketch "Boceto1 (4)" along normal blind 3.13 separate body contours L0 L1 L2 L3 L4 L5 picked at (0.625, -1.082532) makes body 25 in component "Component"
sketch "Boceto2 (4)" plane through (0, 0, 0) normal (0, 0, 1) x (1, 0, 0) in component "Component"
  circle A0 centre (0, 0) radius 2.5
extrude "Extruir2''''" add sketch "Boceto2 (4)" along normal blind 11.5 contours A0 picked at (-0.886301, 0.232065) bodies 25 in component "Component"
chamfer "Chaflán1" distance 0.38 angle 45 1 edges at (-2.330818, -0.904039, 11.5) on bodies 25 in component "Component"
fillet "Empalme1" radius 0.3 1 edges at (-2.330818, 0.904039, 3.13) on bodies 25 in component "Component"
sketch "Boceto3 (5)" plane through (0, 0, 0) normal (0, 1, 0) x (1, 0, 0) in component "Component"
  line L0 (3.247595, 0) -> (3.75, 0)
  line L1 (3.75, 0) -> (3.75, -0.290064)
  line L2 (3.75, -0.290064) -> (3.247595, 0)
sketch "Boceto4 (2)" plane through (0, 0, 0) normal (0, 1, 0) x (1, 0, 0) in component "Component"
  line L0 (3.247595, -3.13) -> (3.75, -3.13)
  line L1 (3.75, -3.13) -> (3.75, -2.839936)
  line L2 (3.75, -2.839936) -> (3.247595, -3.13)
revolve "Revolución1" cut sketch "Boceto4 (2)" angle 360 about axis through (0, 0, 1.75) along (0, 0, 1) contours L0 L1 L2 picked at (3.582532, -3.033312) bodies 25 in component "Component"
revolve "Revolución2" cut sketch "Boceto3 (5)" angle 360 about axis through (0, 0, 1.75) along (0, 0, 1) contours L0 L1 L2 picked at (3.582532, -0.096688) bodies 25 in component "Component"
thread "Rosca1" "ISO Metric profile 0.8 M0.8x0.2 6g" major diameter 0.785 minor diameter 0.54 pitch 0.2 angle 60 resizes the face on face at (2.487577, 0.24892, 5.993333) on bodies 25 in component "Component"
sketch "Boceto12" plane through (-2.8125, -1.623798, 0) normal (-0.8660254, -0.5, 0) x (0.5, -0.8660254, 0)
  spline S0 degree 2 poles (-1.875, 0.290064) (-0.870191, 0) (0, 0) knots 0 0 0 0.19021481 0.19021481 0.19021481 weights 1 1.03795485 1
  spline S1 degree 2 poles (0, 0) (0.870191, 0) (1.875, 0.290064) knots 0.19021481 0.19021481 0.19021481 0.38042962 0.38042962 0.38042962 weights 1 1.03795485 1
  line L0 (1.875, 0.290064) -> (1.875, 2.839936)
  spline S2 degree 2 poles (1.875, 2.839936) (0.870191, 3.13) (0, 3.13) knots 0 0 0 0.19021481 0.19021481 0.19021481 weights 1 1.03795485 1
  spline S3 degree 2 poles (0, 3.13) (-0.870191, 3.13) (-1.875, 2.839936) knots 0.19021481 0.19021481 0.19021481 0.38042962 0.38042962 0.38042962 weights 1 1.03795485 1
  line L1 (-1.875, 2.839936) -> (-1.875, 0.290064)
  line L2 (-3.75, 3.160795) -> (4.229553, 3.160795)
  line L3 (4.229553, 3.160795) -> (4.229553, 0)
  line L4 (4.229553, 0) -> (-3.75, 0)
  line L5 (-3.75, 0) -> (-3.75, 3.160795)
  constraint horizontal L2
  constraint vertical L3
  constraint horizontal L4
  constraint vertical L5
extrude "Extruir3''" cut sketch "Boceto12" against normal blind 7.5 contours S0 S1 L0 S2 S3 L1 | L2 L3 L4 L5 picked at (-1.365055, 1.127055) picked at (3.444702, 2.000244) bodies 25 in component "Component"
move_body "Desplazar1" bodies 25 to x (1, 0, 0) y (0, 0, 1) z (0, -1, 0) at (0, 39.552772, 15.468329) in component "Component"
sketch "Boceto1 (5)" plane through (0, 0, 0) normal (0, 0, 1) x (1, 0, 0) in component "Component'"
  line L0 (1.875, 3.247595) -> (3.75, 0)
  line L1 (-1.875, 3.247595) -> (1.875, 3.247595)
  line L2 (-3.75, 0) -> (-1.875, 3.247595)
  line L3 (-1.875, -3.247595) -> (-3.75, 0)
  line L4 (1.875, -3.247595) -> (-1.875, -3.247595)
  line L5 (3.75, 0) -> (1.875, -3.247595)
extrude "Extruir1'''''" add sketch "Boceto1 (5)" along normal blind 3.13 separate body contours L0 L1 L2 L3 L4 L5 picked at (0.625, -1.082532) makes body 26 in component "Component'"
sketch "Boceto2 (5)" plane through (0, 0, 0) normal (0, 0, 1) x (1, 0, 0) in component "Component'"
  circle A0 centre (0, 0) radius 0.421634
extrude "Extruir2'''''" add sketch "Boceto2 (5)" along normal blind 11.5 contours A0 picked at (0.289422, -0.105292) bodies 26 in component "Component'"
chamfer "Chaflán1'" distance 0.38 angle 45 1 edges at (-0.393101, -0.152469, 11.5) on bodies 26 in component "Component'"
fillet "Empalme1'" radius 0.3 1 edges at (-0.393101, 0.152469, 3.13) on bodies 26 in component "Component'"
sketch "Boceto3 (6)" plane through (0, 0, 0) normal (0, 1, 0) x (1, 0, 0) in component "Component'"
  line L0 (3.247595, 0) -> (3.75, 0)
  line L1 (3.75, 0) -> (3.75, -0.290064)
  line L2 (3.75, -0.290064) -> (3.247595, 0)
sketch "Boceto4 (3)" plane through (0, 0, 0) normal (0, 1, 0) x (1, 0, 0) in component "Component'"
  line L0 (3.247595, -3.13) -> (3.75, -3.13)
  line L1 (3.75, -3.13) -> (3.75, -2.839936)
  line L2 (3.75, -2.839936) -> (3.247595, -3.13)
revolve "Revolución1'" cut sketch "Boceto4 (3)" angle 360 about axis through (0, 0, 2.25) along (0, 0, -1) contours L0 L1 L2 picked at (3.582532, -3.033312) sketch seen with x (-0.15389644, 0.98808698, 0) y (0.98808698, 0.15389644, 0) z (0, 0, -1) at (0, 0, 4) bodies 23 in component "Spur Gear (10 teeth)"
revolve "Revolución1''" cut sketch "Boceto4 (3)" angle 360 about axis through (0, 0, 1.75) along (0, 0, 1) contours L0 L1 L2 picked at (3.582532, -3.033312) bodies 26 in component "Component'"
revolve "Revolución2'" cut sketch "Boceto3 (6)" angle 360 about axis through (0, 0, 1.75) along (0, 0, 1) contours L0 L1 L2 picked at (3.582532, -0.096688) bodies 26 in component "Component'"
thread "Rosca1'" "ISO Metric profile 0.9 M0.9x0.225 6g" major diameter 0.8835 minor diameter 0.608 pitch 0.225 angle 60 resizes the face on face at (0.419539, 0.041981, 5.993333) on bodies 26 in component "Component'"
sketch "Boceto13" plane through (-2.8125, 1.623798, 0) normal (-0.8660254, 0.5, 0) x (-0.5, -0.8660254, 0)
  spline S0 degree 2 poles (-1.875, 0.290064) (-0.870191, 0) (0, 0) knots 0 0 0 0.19021481 0.19021481 0.19021481 weights 1 1.03795485 1
  spline S1 degree 2 poles (0, 0) (0.870191, 0) (1.875, 0.290064) knots 0.19021481 0.19021481 0.19021481 0.38042962 0.38042962 0.38042962 weights 1 1.03795485 1
  line L0 (1.875, 0.290064) -> (1.875, 2.839936)
  spline S2 degree 2 poles (1.875, 2.839936) (0.870191, 3.13) (0, 3.13) knots 0 0 0 0.19021481 0.19021481 0.19021481 weights 1 1.03795485 1
  spline S3 degree 2 poles (0, 3.13) (-0.870191, 3.13) (-1.875, 2.839936) knots 0.19021481 0.19021481 0.19021481 0.38042962 0.38042962 0.38042962 weights 1 1.03795485 1
  line L1 (-1.875, 2.839936) -> (-1.875, 0.290064)
  line L2 (-3.923794, 3.13) -> (4.5, 3.13)
  line L3 (4.5, 3.13) -> (4.5, 0)
  line L4 (4.5, 0) -> (-3.923794, 0)
  line L5 (-3.923794, 0) -> (-3.923794, 3.13)
  constraint horizontal L2
  constraint vertical L3
  constraint horizontal L4
  constraint vertical L5
extrude "Extruir3'''" cut sketch "Boceto13" against normal blind 17.5 contours S0 S1 L0 S2 S3 L1 | S0 S3 L1 L2 L4 L5 | S1 L0 S2 L2 L3 L4 picked at (-1.365055, 1.127055) picked at (-3.240863, 1.140021) picked at (3.625, 1.140021) bodies 26 in component "Component'"
move_body "Desplazar1'" bodies 26 to x (1, 0, 0) y (0, -0.25881905, 0.96592583) z (0, -0.96592583, -0.25881905) at (27.365411, 16.166146, 10.64102) in component "Component'"
ref_plane "PlanoDeObra3" through (12.493594, 8.471695, 21) normal (0, 0, 1) x (0.44467995, 0.89568954, 0)
sketch "Boceto1 (6)" plane through (0, 0, 21) normal (0, 0, 1) x (1, 0, 0) in component "Component''"
  circle A0 centre (12.332883, 8.53815) radius 7.288702
  line L0 (12.290696, 1.24957) -> (12.290696, 15.82673)
  point P0 (12.332883, 8.53815)
  constraint vertical L0
extrude "Extruir1''''''" add sketch "Boceto1 (6)" along normal blind 1 separate body contours A0 L0 picked at (13.610744, 10.586856) makes body 27 in component "Component''"
sketch "Boceto2 (6)" plane through (0, 0, 21) normal (0, 0, -1) x (1, 0, 0) in component "Component''"
  arc A0 (12.290696, -15.82673) -> (12.290696, -1.24957) centre (12.332883, -8.53815) ccw
  line L0 (12.290696, -1.24957) -> (12.290696, -15.82673)
  line L1 (13.503159, -3.968848) -> (12.641027, -3.968848)
  line L2 (12.641027, -3.968848) -> (12.641027, -2.660375)
  line L3 (12.641027, -2.660375) -> (13.503159, -2.660375)
  line L4 (13.503159, -2.660375) -> (13.503159, -3.968848)
  line L5 (13.503159, -14.414887) -> (12.641027, -14.414887)
  line L6 (12.641027, -14.414887) -> (12.641027, -13.097477)
  line L7 (12.641027, -13.097477) -> (13.503159, -13.097477)
  line L8 (13.503159, -13.097477) -> (13.503159, -14.414887)
  point P0 (13.503159, -3.968848)
  constraint horizontal L1
  constraint vertical L2
  constraint horizontal L3
  constraint vertical L4
  constraint horizontal L5
  constraint vertical L6
  constraint horizontal L7
  constraint vertical L8
extrude "Extruir2''''''" add sketch "Boceto2 (6)" along normal blind 2 contours L1 L2 L3 L4 | L5 L6 L7 L8 picked at (13.215782, -3.53269) picked at (13.215782, -13.97575) bodies 27 in component "Component''"
sketch "Boceto3 (7)" plane through (13.503159, 0, 0) normal (1, 0, 0) x (0, 1, 0) in component "Component''"
  line L0 (3.968848, 21) -> (2.660375, 21)
  line L1 (2.660375, 21) -> (2.660375, 19)
  line L2 (2.660375, 19) -> (3.968848, 19)
  line L3 (3.968848, 19) -> (3.968848, 21)
  circle A0 centre (13.8, 19.7) radius 0.5
  circle A1 centre (3.367061, 19.736673) radius 0.516897
  ellipse E0 centre (3.427355, 19.75) end of major axis (3.427355, 19.68825) minor radius 0.06175
extrude "Extruir3''''" cut sketch "Boceto3 (7)" against normal blind 0.9 contours A0 picked at (13.691756, 19.555662) bodies 27 in component "Component''"